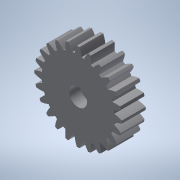
# Autodesk Inventor part: small-gear-v2
Saved by Autodesk Inventor 2020 (Build 240168000, 168)
## iProperties
Created: 2020-08-23
Part Number: small-gear-v2
Material: Ogólny
Document SubType Name: Modeling
Designer: blep
Density: 1 g/cm^3
Appearance: Domyślna
Author: blep
Autodesk Inventor part; units mm, degrees
ref_plane "YZ Plane" through (0, 0, 0) normal (1, 0, 0) x (0, 1, 0)
ref_plane "XZ Plane" through (0, 0, 0) normal (0, 1, 0) x (-1, 0, 0)
ref_plane "XY Plane" through (0, 0, 0) normal (0, 0, 1) x (1, 0, 0)
sketch "Szkic1" plane through (0, 0, 0) normal (0, 0, 1) x (1, 0, 0)
  circle A0 centre (0, 0) radius 10 projected
  arc A1 (-4.8234, -10.5501) -> (-4.0494, -10.8707) centre (0, 0) ccw projected
  arc A2 (-4.0494, -10.8707) -> (-4.0286, -13.3901) centre (5.3777, -12.0526) ccw projected
  arc A3 (-4.0286, -13.3901) -> (-3.2062, -13.6104) centre (0, 0) ccw projected
  arc A4 (-3.2062, -13.6104) -> (-1.9284, -11.439) centre (-10.6836, -7.749) ccw projected
  arc A5 (-1.9284, -11.439) -> (-1.0979, -11.5483) centre (0, 0) ccw projected
  arc A6 (-1.0979, -11.5483) -> (-0.4257, -13.9765) centre (8.3139, -10.2501) ccw projected
  arc A7 (-0.4257, -13.9765) -> (0.4257, -13.9765) centre (0, 0) ccw projected
  arc A8 (0.4257, -13.9765) -> (1.0979, -11.5483) centre (-8.3139, -10.2501) ccw projected
  arc A9 (1.0979, -11.5483) -> (1.9284, -11.439) centre (0, 0) ccw projected
  arc A10 (1.9284, -11.439) -> (3.2062, -13.6104) centre (10.6836, -7.749) ccw projected
  arc A11 (3.2062, -13.6104) -> (4.0286, -13.3901) centre (0, 0) ccw projected
  arc A12 (4.0286, -13.3901) -> (4.0494, -10.8707) centre (-5.3777, -12.0526) ccw projected
  arc A13 (4.0494, -10.8707) -> (4.8234, -10.5501) centre (0, 0) ccw projected
  arc A14 (4.8234, -10.5501) -> (6.6195, -12.3168) centre (12.3251, -4.7199) ccw projected
  arc A15 (6.6195, -12.3168) -> (7.3569, -11.8911) centre (0, 0) ccw projected
  arc A16 (7.3569, -11.8911) -> (6.725, -9.4522) centre (-2.075, -13.0338) ccw projected
  arc A17 (6.725, -9.4522) -> (7.3896, -8.9422) centre (0, 0) ccw projected
  arc A18 (7.3896, -8.9422) -> (9.5818, -10.1839) centre (13.1267, -1.3691) ccw projected
  arc A19 (9.5818, -10.1839) -> (10.1839, -9.5818) centre (0, 0) ccw projected
  arc A20 (10.1839, -9.5818) -> (8.9422, -7.3896) centre (1.3691, -13.1267) ccw projected
  arc A21 (8.9422, -7.3896) -> (9.4522, -6.725) centre (0, 0) ccw projected
  arc A22 (9.4522, -6.725) -> (11.8911, -7.3569) centre (13.0338, 2.075) ccw projected
  arc A23 (11.8911, -7.3569) -> (12.3168, -6.6195) centre (0, 0) ccw projected
  arc A24 (12.3168, -6.6195) -> (10.5501, -4.8234) centre (4.7199, -12.3251) ccw projected
  arc A25 (10.5501, -4.8234) -> (10.8707, -4.0494) centre (0, 0) ccw projected
  arc A26 (10.8707, -4.0494) -> (13.3901, -4.0286) centre (12.0526, 5.3777) ccw projected
  arc A27 (13.3901, -4.0286) -> (13.6104, -3.2062) centre (0, 0) ccw projected
  arc A28 (13.6104, -3.2062) -> (11.439, -1.9284) centre (7.749, -10.6836) ccw projected
  arc A29 (11.439, -1.9284) -> (11.5483, -1.0979) centre (0, 0) ccw projected
  arc A30 (11.5483, -1.0979) -> (13.9765, -0.4257) centre (10.2501, 8.3139) ccw projected
  arc A31 (13.9765, -0.4257) -> (13.9765, 0.4257) centre (0, 0) ccw projected
  arc A32 (13.9765, 0.4257) -> (11.5483, 1.0979) centre (10.2501, -8.3139) ccw projected
  arc A33 (11.5483, 1.0979) -> (11.439, 1.9284) centre (0, 0) ccw projected
  arc A34 (11.439, 1.9284) -> (13.6104, 3.2062) centre (7.749, 10.6836) ccw projected
  arc A35 (13.6104, 3.2062) -> (13.3901, 4.0286) centre (0, 0) ccw projected
  arc A36 (13.3901, 4.0286) -> (10.8707, 4.0494) centre (12.0526, -5.3777) ccw projected
  arc A37 (10.8707, 4.0494) -> (10.5501, 4.8234) centre (0, 0) ccw projected
  arc A38 (10.5501, 4.8234) -> (12.3168, 6.6195) centre (4.7199, 12.3251) ccw projected
  arc A39 (12.3168, 6.6195) -> (11.8911, 7.3569) centre (0, 0) ccw projected
  arc A40 (11.8911, 7.3569) -> (9.4522, 6.725) centre (13.0338, -2.075) ccw projected
  arc A41 (9.4522, 6.725) -> (8.9422, 7.3896) centre (0, 0) ccw projected
  arc A42 (8.9422, 7.3896) -> (10.1839, 9.5818) centre (1.3691, 13.1267) ccw projected
  arc A43 (10.1839, 9.5818) -> (9.5818, 10.1839) centre (0, 0) ccw projected
  arc A44 (9.5818, 10.1839) -> (7.3896, 8.9422) centre (13.1267, 1.3691) ccw projected
  arc A45 (7.3896, 8.9422) -> (6.725, 9.4522) centre (0, 0) ccw projected
  arc A46 (6.725, 9.4522) -> (7.3569, 11.8911) centre (-2.075, 13.0338) ccw projected
  arc A47 (7.3569, 11.8911) -> (6.6195, 12.3168) centre (0, 0) ccw projected
  arc A48 (6.6195, 12.3168) -> (4.8234, 10.5501) centre (12.3251, 4.7199) ccw projected
  arc A49 (4.8234, 10.5501) -> (4.0494, 10.8707) centre (0, 0) ccw projected
  arc A50 (4.0494, 10.8707) -> (4.0286, 13.3901) centre (-5.3777, 12.0526) ccw projected
  arc A51 (4.0286, 13.3901) -> (3.2062, 13.6104) centre (0, 0) ccw projected
  arc A52 (3.2062, 13.6104) -> (1.9284, 11.439) centre (10.6836, 7.749) ccw projected
  arc A53 (1.9284, 11.439) -> (1.0979, 11.5483) centre (0, 0) ccw projected
  arc A54 (1.0979, 11.5483) -> (0.4257, 13.9765) centre (-8.3139, 10.2501) ccw projected
  arc A55 (0.4257, 13.9765) -> (-0.4257, 13.9765) centre (0, 0) ccw projected
  arc A56 (-0.4257, 13.9765) -> (-1.0979, 11.5483) centre (8.3139, 10.2501) ccw projected
  arc A57 (-1.0979, 11.5483) -> (-1.9284, 11.439) centre (0, 0) ccw projected
  arc A58 (-1.9284, 11.439) -> (-3.2062, 13.6104) centre (-10.6836, 7.749) ccw projected
  arc A59 (-3.2062, 13.6104) -> (-4.0286, 13.3901) centre (0, 0) ccw projected
  arc A60 (-4.0286, 13.3901) -> (-4.0494, 10.8707) centre (5.3777, 12.0526) ccw projected
  arc A61 (-4.0494, 10.8707) -> (-4.8234, 10.5501) centre (0, 0) ccw projected
  arc A62 (-4.8234, 10.5501) -> (-6.6195, 12.3168) centre (-12.3251, 4.7199) ccw projected
  arc A63 (-6.6195, 12.3168) -> (-7.3569, 11.8911) centre (0, 0) ccw projected
  arc A64 (-7.3569, 11.8911) -> (-6.725, 9.4522) centre (2.075, 13.0338) ccw projected
  arc A65 (-6.725, 9.4522) -> (-7.3896, 8.9422) centre (0, 0) ccw projected
  arc A66 (-7.3896, 8.9422) -> (-9.5818, 10.1839) centre (-13.1267, 1.3691) ccw projected
  arc A67 (-9.5818, 10.1839) -> (-10.1839, 9.5818) centre (0, 0) ccw projected
  arc A68 (-10.1839, 9.5818) -> (-8.9422, 7.3896) centre (-1.3691, 13.1267) ccw projected
  arc A69 (-8.9422, 7.3896) -> (-9.4522, 6.725) centre (0, 0) ccw projected
  arc A70 (-9.4522, 6.725) -> (-11.8911, 7.3569) centre (-13.0338, -2.075) ccw projected
  arc A71 (-11.8911, 7.3569) -> (-12.3168, 6.6195) centre (0, 0) ccw projected
  arc A72 (-12.3168, 6.6195) -> (-10.5501, 4.8234) centre (-4.7199, 12.3251) ccw projected
  arc A73 (-10.5501, 4.8234) -> (-10.8707, 4.0494) centre (0, 0) ccw projected
  arc A74 (-10.8707, 4.0494) -> (-13.3901, 4.0286) centre (-12.0526, -5.3777) ccw projected
  arc A75 (-13.3901, 4.0286) -> (-13.6104, 3.2062) centre (0, 0) ccw projected
  arc A76 (-13.6104, 3.2062) -> (-11.439, 1.9284) centre (-7.749, 10.6836) ccw projected
  arc A77 (-11.439, 1.9284) -> (-11.5483, 1.0979) centre (0, 0) ccw projected
  arc A78 (-11.5483, 1.0979) -> (-13.9765, 0.4257) centre (-10.2501, -8.3139) ccw projected
  arc A79 (-13.9765, 0.4257) -> (-13.9765, -0.4257) centre (0, 0) ccw projected
  arc A80 (-13.9765, -0.4257) -> (-11.5483, -1.0979) centre (-10.2501, 8.3139) ccw projected
  arc A81 (-11.5483, -1.0979) -> (-11.439, -1.9284) centre (0, 0) ccw projected
  arc A82 (-11.439, -1.9284) -> (-13.6104, -3.2062) centre (-7.749, -10.6836) ccw projected
  arc A83 (-13.6104, -3.2062) -> (-13.3901, -4.0286) centre (0, 0) ccw projected
  arc A84 (-13.3901, -4.0286) -> (-10.8707, -4.0494) centre (-12.0526, 5.3777) ccw projected
  arc A85 (-10.8707, -4.0494) -> (-10.5501, -4.8234) centre (0, 0) ccw projected
  arc A86 (-10.5501, -4.8234) -> (-12.3168, -6.6195) centre (-4.7199, -12.3251) ccw projected
  arc A87 (-12.3168, -6.6195) -> (-11.8911, -7.3569) centre (0, 0) ccw projected
  arc A88 (-11.8911, -7.3569) -> (-9.4522, -6.725) centre (-13.0338, 2.075) ccw projected
  arc A89 (-9.4522, -6.725) -> (-8.9422, -7.3896) centre (0, 0) ccw projected
  arc A90 (-8.9422, -7.3896) -> (-10.1839, -9.5818) centre (-1.3691, -13.1267) ccw projected
  arc A91 (-10.1839, -9.5818) -> (-9.5818, -10.1839) centre (0, 0) ccw projected
  arc A92 (-9.5818, -10.1839) -> (-7.3896, -8.9422) centre (-13.1267, -1.3691) ccw projected
  arc A93 (-7.3896, -8.9422) -> (-6.725, -9.4522) centre (0, 0) ccw projected
  arc A94 (-6.725, -9.4522) -> (-7.3569, -11.8911) centre (2.075, -13.0338) ccw projected
  arc A95 (-7.3569, -11.8911) -> (-6.6195, -12.3168) centre (0, 0) ccw projected
  arc A96 (-6.6195, -12.3168) -> (-4.8234, -10.5501) centre (-12.3251, -4.7199) ccw projected
  point P0 (0, 0)
extrude "Wyciągnięcie proste1" add sketch "Szkic1" along normal blind 7.6 contours A0 | A96 A95 A94 A93 A92 A91 A90 A89 A88 A87 A86 A85 A84 A83 A82 A81 A80 A79 A78 A77 A76 A75 A74 A73 A72 A71 A70 A69 A68 A67 A66 A65 A64 A63 A62 A61 A60 A59 A58 A57 A56 A55 A54 A53 A52 A51 A50 A49 A48 A47 A46 A45 A44 A43 A42 A41 A40 A39 A38 A37 A36 A35 A34 A33 A32 A31 A30 A29 A28 A27 A26 A25 A24 A23 A22 A21 A20 A19 A18 A17 A16 A15 A14 A13 A12 A11 A10 A9 A8 A7 A6 A5 A4 A3 A2 A1
sketch "Szkic2" plane through (0, 0, 7.6) normal (0, 0, 1) x (1, 0, 0)
  circle A0 centre (0, 0) radius 0.8 projected
  line L0 (1.024, 2.4534) -> (1.397, 2.2614) projected
  line L1 (1.397, 2.2614) -> (1.4153, 2.1811) projected
  arc A1 (1.4994, 2.1241) -> (1.4153, 2.1811) centre (0, 0) ccw projected
  line L2 (1.4994, 2.1241) -> (1.5814, 2.137) projected
  line L3 (1.5814, 2.137) -> (1.8976, 1.8613) projected
  line L4 (1.8976, 1.8613) -> (1.8961, 1.779) projected
  arc A2 (1.9642, 1.7035) -> (1.8961, 1.779) centre (0, 0) ccw projected
  line L5 (1.9642, 1.7035) -> (2.0468, 1.6965) projected
  line L6 (2.0468, 1.6965) -> (2.2879, 1.3531) projected
  line L7 (2.2879, 1.3531) -> (2.2668, 1.2735) projected
  arc A3 (2.3148, 1.184) -> (2.2668, 1.2735) centre (0, 0) ccw projected
  line L8 (2.3148, 1.184) -> (2.3934, 1.1574) projected
  line L9 (2.3934, 1.1574) -> (2.5452, 0.7663) projected
  line L10 (2.5452, 0.7663) -> (2.5057, 0.694) projected
  arc A4 (2.5309, 0.5956) -> (2.5057, 0.694) centre (0, 0) ccw projected
  line L11 (2.5309, 0.5956) -> (2.6008, 0.551) projected
  line L12 (2.6008, 0.551) -> (2.6546, 0.1349) projected
  line L13 (2.6546, 0.1349) -> (2.5989, 0.0742) projected
  arc A5 (2.5999, -0.0274) -> (2.5989, 0.0742) centre (0, 0) ccw projected
  line L14 (2.5999, -0.0274) -> (2.6571, -0.0875) projected
  line L15 (2.6571, -0.0875) -> (2.6098, -0.5043) projected
  line L16 (2.6098, -0.5043) -> (2.5412, -0.5499) projected
  arc A6 (2.5178, -0.6487) -> (2.5412, -0.5499) centre (0, 0) ccw projected
  line L17 (2.5178, -0.6487) -> (2.5589, -0.7208) projected
  line L18 (2.5589, -0.7208) -> (2.4133, -1.1142) projected
  line L19 (2.4133, -1.1142) -> (2.3357, -1.1421) projected
  arc A7 (2.2893, -1.2324) -> (2.3357, -1.1421) centre (0, 0) ccw projected
  line L20 (2.2893, -1.2324) -> (2.3121, -1.3122) projected
  line L21 (2.3121, -1.3122) -> (2.0765, -1.6594) projected
  line L22 (2.0765, -1.6594) -> (1.9946, -1.6679) projected
  arc A8 (1.9279, -1.7445) -> (1.9946, -1.6679) centre (0, 0) ccw projected
  line L23 (1.9279, -1.7445) -> (1.9309, -1.8274) projected
  line L24 (1.9309, -1.8274) -> (1.619, -2.1081) projected
  line L25 (1.619, -2.1081) -> (1.5375, -2.0967) projected
  arc A9 (1.4544, -2.1552) -> (1.5375, -2.0967) centre (0, 0) ccw projected
  line L26 (1.4544, -2.1552) -> (1.4374, -2.2364) projected
  line L27 (1.4374, -2.2364) -> (1.0675, -2.4343) projected
  line L28 (1.0675, -2.4343) -> (0.991, -2.4037) projected
  arc A10 (0.8963, -2.4406) -> (0.991, -2.4037) centre (0, 0) ccw projected
  line L29 (0.8963, -2.4406) -> (0.8604, -2.5154) projected
  line L30 (0.8604, -2.5154) -> (0.4539, -2.619) projected
  line L31 (0.4539, -2.619) -> (0.387, -2.571) projected
  arc A11 (0.2862, -2.5842) -> (0.387, -2.571) centre (0, 0) ccw projected
  line L32 (0.2862, -2.5842) -> (0.2335, -2.6482) projected
  line L33 (0.2335, -2.6482) -> (-0.1861, -2.6515) projected
  line L34 (-0.1861, -2.6515) -> (-0.2396, -2.5889) projected
  arc A12 (-0.3405, -2.5776) -> (-0.2396, -2.5889) centre (0, 0) ccw projected
  line L35 (-0.3405, -2.5776) -> (-0.4071, -2.6272) projected
  line L36 (-0.4071, -2.6272) -> (-0.8152, -2.53) projected
  line L37 (-0.8152, -2.53) -> (-0.8522, -2.4564) projected
  arc A13 (-0.9475, -2.4212) -> (-0.8522, -2.4564) centre (0, 0) ccw projected
  line L38 (-0.9475, -2.4212) -> (-1.024, -2.4534) projected
  line L39 (-1.024, -2.4534) -> (-1.397, -2.2614) projected
  line L40 (-1.397, -2.2614) -> (-1.4153, -2.1811) projected
  arc A14 (-1.4994, -2.1241) -> (-1.4153, -2.1811) centre (0, 0) ccw projected
  line L41 (-1.4994, -2.1241) -> (-1.5814, -2.137) projected
  line L42 (-1.5814, -2.137) -> (-1.8976, -1.8613) projected
  line L43 (-1.8976, -1.8613) -> (-1.8961, -1.779) projected
  arc A15 (-1.9642, -1.7035) -> (-1.8961, -1.779) centre (0, 0) ccw projected
  line L44 (-1.9642, -1.7035) -> (-2.0468, -1.6965) projected
  line L45 (-2.0468, -1.6965) -> (-2.2879, -1.3531) projected
  line L46 (-2.2879, -1.3531) -> (-2.2668, -1.2735) projected
  arc A16 (-2.3148, -1.184) -> (-2.2668, -1.2735) centre (0, 0) ccw projected
  line L47 (-2.3148, -1.184) -> (-2.3934, -1.1574) projected
  line L48 (-2.3934, -1.1574) -> (-2.5452, -0.7663) projected
  line L49 (-2.5452, -0.7663) -> (-2.5057, -0.694) projected
  arc A17 (-2.5309, -0.5956) -> (-2.5057, -0.694) centre (0, 0) ccw projected
  line L50 (-2.5309, -0.5956) -> (-2.6008, -0.551) projected
  line L51 (-2.6008, -0.551) -> (-2.6546, -0.1349) projected
  line L52 (-2.6546, -0.1349) -> (-2.5989, -0.0742) projected
  arc A18 (-2.5999, 0.0274) -> (-2.5989, -0.0742) centre (0, 0) ccw projected
  line L53 (-2.5999, 0.0274) -> (-2.6571, 0.0875) projected
  line L54 (-2.6571, 0.0875) -> (-2.6098, 0.5043) projected
  line L55 (-2.6098, 0.5043) -> (-2.5412, 0.5499) projected
  arc A19 (-2.5178, 0.6487) -> (-2.5412, 0.5499) centre (0, 0) ccw projected
  line L56 (-2.5178, 0.6487) -> (-2.5589, 0.7208) projected
  line L57 (-2.5589, 0.7208) -> (-2.4133, 1.1142) projected
  line L58 (-2.4133, 1.1142) -> (-2.3357, 1.1421) projected
  arc A20 (-2.2893, 1.2324) -> (-2.3357, 1.1421) centre (0, 0) ccw projected
  line L59 (-2.2893, 1.2324) -> (-2.3121, 1.3122) projected
  line L60 (-2.3121, 1.3122) -> (-2.0765, 1.6594) projected
  line L61 (-2.0765, 1.6594) -> (-1.9946, 1.6679) projected
  arc A21 (-1.9279, 1.7445) -> (-1.9946, 1.6679) centre (0, 0) ccw projected
  line L62 (-1.9279, 1.7445) -> (-1.9309, 1.8274) projected
  line L63 (-1.9309, 1.8274) -> (-1.619, 2.1081) projected
  line L64 (-1.619, 2.1081) -> (-1.5375, 2.0967) projected
  arc A22 (-1.4544, 2.1552) -> (-1.5375, 2.0967) centre (0, 0) ccw projected
  line L65 (-1.4544, 2.1552) -> (-1.4374, 2.2364) projected
  line L66 (-1.4374, 2.2364) -> (-1.0675, 2.4343) projected
  line L67 (-1.0675, 2.4343) -> (-0.991, 2.4037) projected
  arc A23 (-0.8963, 2.4406) -> (-0.991, 2.4037) centre (0, 0) ccw projected
  line L68 (-0.8963, 2.4406) -> (-0.8604, 2.5154) projected
  line L69 (-0.8604, 2.5154) -> (-0.4539, 2.619) projected
  line L70 (-0.4539, 2.619) -> (-0.387, 2.571) projected
  arc A24 (-0.2862, 2.5842) -> (-0.387, 2.571) centre (0, 0) ccw projected
  line L71 (-0.2862, 2.5842) -> (-0.2335, 2.6482) projected
  line L72 (-0.2335, 2.6482) -> (0.1861, 2.6515) projected
  line L73 (0.1861, 2.6515) -> (0.2396, 2.5889) projected
  arc A25 (0.3405, 2.5776) -> (0.2396, 2.5889) centre (0, 0) ccw projected
  line L74 (0.3405, 2.5776) -> (0.4071, 2.6272) projected
  line L75 (0.4071, 2.6272) -> (0.8152, 2.53) projected
  line L76 (0.8152, 2.53) -> (0.8522, 2.4564) projected
  arc A26 (0.9475, 2.4212) -> (0.8522, 2.4564) centre (0, 0) ccw projected
  line L77 (0.9475, 2.4212) -> (1.024, 2.4534) projected
  line L78 (-2.8819, 0.3236) -> (-2.6571, 0.0875) projected
  line L79 (-2.6098, 0.5043) -> (-2.8819, 0.3236) projected
  line L80 (-2.6571, 0.0875) -> (-2.6098, 0.5043) projected
  line L81 (-2.8819, 0.3236) -> (-2.6571, 0.0875) projected
  circle A27 centre (0, 0) radius 2.85
  point P0 (0, 0)
  point P1 (-2.8366, 0.276)
  point P2 (-2.8272, 0.3599)
  dimension "d2" = 5.7
  constraints: 1 centre point, 1 coincident
  measures "d2" diameter of A27
extrude "Wyciągnięcie proste2" cut sketch "Szkic2" against normal blind 3.5 contours A0 | L77 A26 L76 L75 L74 A25 L73 L72 L71 A24 L70 L69 L68 A23 L67 L66 L65 A22 L64 L63 L62 A21 L61 L60 L59 A20 L58 L57 L56 A19 L55 L79 A27 L78 L53 A18 L52 L51 L50 A17 L49 L48 L47 A16 L46 L45 L44 A15 L43 L42 L41 A14 L40 L39 L38 A13 L37 L36 L35 A12 L34 L33 L32 A11 L31 L30 L29 A10 L28 L27 L26 A9 L25 L24 L23 A8 L22 L21 L20 A7 L19 L18 L17 A6 L16 L15 L14 A5 L13 L12 L11 A4 L10 L9 L8 A3 L7 L6 L5 A2 L4 L3 L2 A1 L1 L0 | L0 L1 A1 L2 L3 L4 A2 L5 L6 L7 A3 L8 L9 L10 A4 L11 L12 L13 A5 L14 L15 L16 A6 L17 L18 L19 A7 L20 L21 L22 A8 L23 L24 L25 A9 L26 L27 L28 A10 L29 L30 L31 A11 L32 L33 L34 A12 L35 L36 L37 A13 L38 L39 L40 A14 L41 L42 L43 A15 L44 L45 L46 A16 L47 L48 L49 A17 L50 L51 L52 A18 L53 L54 L55 A19 L56 L57 L58 A20 L59 L60 L61 A21 L62 L63 L64 A22 L65 L66 L67 A23 L68 L69 L70 A24 L71 L72 L73 A25 L74 L75 L76 A26 L77 | L54 L78 A27 L79
sketch "Szkic3" plane through (0, 0, 7.6) normal (0, 0, 1) x (1, 0, 0)
  circle A0 centre (0, 0) radius 0.8 projected
  point P0 (0, 0)
extrude "Wyciągnięcie proste3" cut sketch "Szkic3" against normal through all
sketch "Szkic5" plane through (0, 0, 0) normal (0, 0, -1) x (-1, 0, 0)
  circle A0 centre (0, 0) radius 2.85 projected
  arc A1 (-6.6195, -12.3168) -> (-4.8234, -10.5501) centre (-12.3251, -4.7199) ccw projected
  arc A2 (-7.3569, -11.8911) -> (-6.6195, -12.3168) centre (0, 0) ccw projected
  arc A3 (-6.725, -9.4522) -> (-7.3569, -11.8911) centre (2.075, -13.0338) ccw projected
  arc A4 (-7.3896, -8.9422) -> (-6.725, -9.4522) centre (0, 0) ccw projected
  arc A5 (-9.5818, -10.1839) -> (-7.3896, -8.9422) centre (-13.1267, -1.3691) ccw projected
  arc A6 (-10.1839, -9.5818) -> (-9.5818, -10.1839) centre (0, 0) ccw projected
  arc A7 (-8.9422, -7.3896) -> (-10.1839, -9.5818) centre (-1.3691, -13.1267) ccw projected
  arc A8 (-9.4522, -6.725) -> (-8.9422, -7.3896) centre (0, 0) ccw projected
  arc A9 (-11.8911, -7.3569) -> (-9.4522, -6.725) centre (-13.0338, 2.075) ccw projected
  arc A10 (-12.3168, -6.6195) -> (-11.8911, -7.3569) centre (0, 0) ccw projected
  arc A11 (-10.5501, -4.8234) -> (-12.3168, -6.6195) centre (-4.7199, -12.3251) ccw projected
  arc A12 (-10.8707, -4.0494) -> (-10.5501, -4.8234) centre (0, 0) ccw projected
  arc A13 (-13.3901, -4.0286) -> (-10.8707, -4.0494) centre (-12.0526, 5.3777) ccw projected
  arc A14 (-13.6104, -3.2062) -> (-13.3901, -4.0286) centre (0, 0) ccw projected
  arc A15 (-11.439, -1.9284) -> (-13.6104, -3.2062) centre (-7.749, -10.6836) ccw projected
  arc A16 (-11.5483, -1.0979) -> (-11.439, -1.9284) centre (0, 0) ccw projected
  arc A17 (-13.9765, -0.4257) -> (-11.5483, -1.0979) centre (-10.2501, 8.3139) ccw projected
  arc A18 (-13.9765, 0.4257) -> (-13.9765, -0.4257) centre (0, 0) ccw projected
  arc A19 (-11.5483, 1.0979) -> (-13.9765, 0.4257) centre (-10.2501, -8.3139) ccw projected
  arc A20 (-11.439, 1.9284) -> (-11.5483, 1.0979) centre (0, 0) ccw projected
  arc A21 (-13.6104, 3.2062) -> (-11.439, 1.9284) centre (-7.749, 10.6836) ccw projected
  arc A22 (-13.3901, 4.0286) -> (-13.6104, 3.2062) centre (0, 0) ccw projected
  arc A23 (-10.8707, 4.0494) -> (-13.3901, 4.0286) centre (-12.0526, -5.3777) ccw projected
  arc A24 (-10.5501, 4.8234) -> (-10.8707, 4.0494) centre (0, 0) ccw projected
  arc A25 (-12.3168, 6.6195) -> (-10.5501, 4.8234) centre (-4.7199, 12.3251) ccw projected
  arc A26 (-11.8911, 7.3569) -> (-12.3168, 6.6195) centre (0, 0) ccw projected
  arc A27 (-9.4522, 6.725) -> (-11.8911, 7.3569) centre (-13.0338, -2.075) ccw projected
  arc A28 (-8.9422, 7.3896) -> (-9.4522, 6.725) centre (0, 0) ccw projected
  arc A29 (-10.1839, 9.5818) -> (-8.9422, 7.3896) centre (-1.3691, 13.1267) ccw projected
  arc A30 (-9.5818, 10.1839) -> (-10.1839, 9.5818) centre (0, 0) ccw projected
  arc A31 (-7.3896, 8.9422) -> (-9.5818, 10.1839) centre (-13.1267, 1.3691) ccw projected
  arc A32 (-6.725, 9.4522) -> (-7.3896, 8.9422) centre (0, 0) ccw projected
  arc A33 (-7.3569, 11.8911) -> (-6.725, 9.4522) centre (2.075, 13.0338) ccw projected
  arc A34 (-6.6195, 12.3168) -> (-7.3569, 11.8911) centre (0, 0) ccw projected
  arc A35 (-4.8234, 10.5501) -> (-6.6195, 12.3168) centre (-12.3251, 4.7199) ccw projected
  arc A36 (-4.0494, 10.8707) -> (-4.8234, 10.5501) centre (0, 0) ccw projected
  arc A37 (-4.0286, 13.3901) -> (-4.0494, 10.8707) centre (5.3777, 12.0526) ccw projected
  arc A38 (-3.2062, 13.6104) -> (-4.0286, 13.3901) centre (0, 0) ccw projected
  arc A39 (-1.9284, 11.439) -> (-3.2062, 13.6104) centre (-10.6836, 7.749) ccw projected
  arc A40 (-1.0979, 11.5483) -> (-1.9284, 11.439) centre (0, 0) ccw projected
  arc A41 (-0.4257, 13.9765) -> (-1.0979, 11.5483) centre (8.3139, 10.2501) ccw projected
  arc A42 (0.4257, 13.9765) -> (-0.4257, 13.9765) centre (0, 0) ccw projected
  arc A43 (1.0979, 11.5483) -> (0.4257, 13.9765) centre (-8.3139, 10.2501) ccw projected
  arc A44 (1.9284, 11.439) -> (1.0979, 11.5483) centre (0, 0) ccw projected
  arc A45 (3.2062, 13.6104) -> (1.9284, 11.439) centre (10.6836, 7.749) ccw projected
  arc A46 (4.0286, 13.3901) -> (3.2062, 13.6104) centre (0, 0) ccw projected
  arc A47 (4.0494, 10.8707) -> (4.0286, 13.3901) centre (-5.3777, 12.0526) ccw projected
  arc A48 (4.8234, 10.5501) -> (4.0494, 10.8707) centre (0, 0) ccw projected
  arc A49 (6.6195, 12.3168) -> (4.8234, 10.5501) centre (12.3251, 4.7199) ccw projected
  arc A50 (7.3569, 11.8911) -> (6.6195, 12.3168) centre (0, 0) ccw projected
  arc A51 (6.725, 9.4522) -> (7.3569, 11.8911) centre (-2.075, 13.0338) ccw projected
  arc A52 (7.3896, 8.9422) -> (6.725, 9.4522) centre (0, 0) ccw projected
  arc A53 (9.5818, 10.1839) -> (7.3896, 8.9422) centre (13.1267, 1.3691) ccw projected
  arc A54 (10.1839, 9.5818) -> (9.5818, 10.1839) centre (0, 0) ccw projected
  arc A55 (8.9422, 7.3896) -> (10.1839, 9.5818) centre (1.3691, 13.1267) ccw projected
  arc A56 (9.4522, 6.725) -> (8.9422, 7.3896) centre (0, 0) ccw projected
  arc A57 (11.8911, 7.3569) -> (9.4522, 6.725) centre (13.0338, -2.075) ccw projected
  arc A58 (12.3168, 6.6195) -> (11.8911, 7.3569) centre (0, 0) ccw projected
  arc A59 (10.5501, 4.8234) -> (12.3168, 6.6195) centre (4.7199, 12.3251) ccw projected
  arc A60 (10.8707, 4.0494) -> (10.5501, 4.8234) centre (0, 0) ccw projected
  arc A61 (13.3901, 4.0286) -> (10.8707, 4.0494) centre (12.0526, -5.3777) ccw projected
  arc A62 (13.6104, 3.2062) -> (13.3901, 4.0286) centre (0, 0) ccw projected
  arc A63 (11.439, 1.9284) -> (13.6104, 3.2062) centre (7.749, 10.6836) ccw projected
  arc A64 (11.5483, 1.0979) -> (11.439, 1.9284) centre (0, 0) ccw projected
  arc A65 (13.9765, 0.4257) -> (11.5483, 1.0979) centre (10.2501, -8.3139) ccw projected
  arc A66 (13.9765, -0.4257) -> (13.9765, 0.4257) centre (0, 0) ccw projected
  arc A67 (11.5483, -1.0979) -> (13.9765, -0.4257) centre (10.2501, 8.3139) ccw projected
  arc A68 (11.439, -1.9284) -> (11.5483, -1.0979) centre (0, 0) ccw projected
  arc A69 (13.6104, -3.2062) -> (11.439, -1.9284) centre (7.749, -10.6836) ccw projected
  arc A70 (13.3901, -4.0286) -> (13.6104, -3.2062) centre (0, 0) ccw projected
  arc A71 (10.8707, -4.0494) -> (13.3901, -4.0286) centre (12.0526, 5.3777) ccw projected
  arc A72 (10.5501, -4.8234) -> (10.8707, -4.0494) centre (0, 0) ccw projected
  arc A73 (12.3168, -6.6195) -> (10.5501, -4.8234) centre (4.7199, -12.3251) ccw projected
  arc A74 (11.8911, -7.3569) -> (12.3168, -6.6195) centre (0, 0) ccw projected
  arc A75 (9.4522, -6.725) -> (11.8911, -7.3569) centre (13.0338, 2.075) ccw projected
  arc A76 (8.9422, -7.3896) -> (9.4522, -6.725) centre (0, 0) ccw projected
  arc A77 (10.1839, -9.5818) -> (8.9422, -7.3896) centre (1.3691, -13.1267) ccw projected
  arc A78 (9.5818, -10.1839) -> (10.1839, -9.5818) centre (0, 0) ccw projected
  arc A79 (7.3896, -8.9422) -> (9.5818, -10.1839) centre (13.1267, -1.3691) ccw projected
  arc A80 (6.725, -9.4522) -> (7.3896, -8.9422) centre (0, 0) ccw projected
  arc A81 (7.3569, -11.8911) -> (6.725, -9.4522) centre (-2.075, -13.0338) ccw projected
  arc A82 (6.6195, -12.3168) -> (7.3569, -11.8911) centre (0, 0) ccw projected
  arc A83 (4.8234, -10.5501) -> (6.6195, -12.3168) centre (12.3251, -4.7199) ccw projected
  arc A84 (4.0494, -10.8707) -> (4.8234, -10.5501) centre (0, 0) ccw projected
  arc A85 (4.0286, -13.3901) -> (4.0494, -10.8707) centre (-5.3777, -12.0526) ccw projected
  arc A86 (3.2062, -13.6104) -> (4.0286, -13.3901) centre (0, 0) ccw projected
  arc A87 (1.9284, -11.439) -> (3.2062, -13.6104) centre (10.6836, -7.749) ccw projected
  arc A88 (1.0979, -11.5483) -> (1.9284, -11.439) centre (0, 0) ccw projected
  arc A89 (0.4257, -13.9765) -> (1.0979, -11.5483) centre (-8.3139, -10.2501) ccw projected
  arc A90 (-0.4257, -13.9765) -> (0.4257, -13.9765) centre (0, 0) ccw projected
  arc A91 (-1.0979, -11.5483) -> (-0.4257, -13.9765) centre (8.3139, -10.2501) ccw projected
  arc A92 (-1.9284, -11.439) -> (-1.0979, -11.5483) centre (0, 0) ccw projected
  arc A93 (-3.2062, -13.6104) -> (-1.9284, -11.439) centre (-10.6836, -7.749) ccw projected
  arc A94 (-4.0286, -13.3901) -> (-3.2062, -13.6104) centre (0, 0) ccw projected
  arc A95 (-4.0494, -10.8707) -> (-4.0286, -13.3901) centre (5.3777, -12.0526) ccw projected
  arc A96 (-4.8234, -10.5501) -> (-4.0494, -10.8707) centre (0, 0) ccw projected
  point P0 (0, 0)
extrude "Wyciągnięcie proste5" cut sketch "Szkic5" against normal blind 2 contours A0
